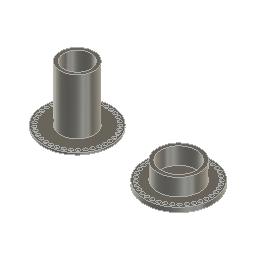
Drum (Autodesk Fusion 360 design; units mm, degrees)
part number: 2026-02-25-13-37-31-976
Autodesk Fusion 360 part; units mm, degrees
note: some values were not read from the file. Chosen so that the rebuilt part matches the saved one: which face or edge a step refers to.
sketch "Sketch1" plane through (0, 0, 0) normal (0, 0, 1) x (1, 0, 0)
  circle A0 centre (0, 0) radius 20
  circle A1 centre (-48, 22) radius 1.1
  dimension "d1" = 40
  dimension "d2" = 2.2
  constraint coincident A0.centre origin
  measures "d1" diameter of A0
  measures "d2" diameter of A1
extrude "Extrude1" add sketch "Sketch1" along normal blind 1.25 contours A0 makes body 1
sketch "Sketch2" plane through (0, 0, 1.25) normal (0, 0, 1) x (-1, 0, 0)
  circle A0 centre (0, 0) radius 20
  circle A1 centre (18, 0) radius 1.1
  circle A2 centre (17.7411, 3.042) radius 1.1
  circle A3 centre (16.9718, 5.9965) radius 1.1
  circle A4 centre (15.7143, 8.7785) radius 1.1
  circle A5 centre (14.0046, 11.308) radius 1.1
  circle A6 centre (11.8921, 13.5121) radius 1.1
  circle A7 centre (9.4375, 15.3275) radius 1.1
  circle A8 centre (6.7114, 16.702) radius 1.1
  circle A9 centre (3.7922, 17.596) radius 1.1
  circle A10 centre (0.7639, 17.9838) radius 1.1
  circle A11 centre (-2.2863, 17.8542) radius 1.1
  circle A12 centre (-5.2708, 17.211) radius 1.1
  circle A13 centre (-8.1037, 16.0727) radius 1.1
  circle A14 centre (-10.7034, 14.4719) radius 1.1
  circle A15 centre (-12.9952, 12.4549) radius 1.1
  circle A16 centre (-14.9132, 10.0795) radius 1.1
  circle A17 centre (-16.4021, 7.4142) radius 1.1
  circle A18 centre (-17.4192, 4.5356) radius 1.1
  circle A19 centre (-17.9352, 1.5265) radius 1.1
  circle A20 centre (-17.9352, -1.5265) radius 1.1
  circle A21 centre (-17.4192, -4.5356) radius 1.1
  circle A22 centre (-16.4021, -7.4142) radius 1.1
  circle A23 centre (-14.9132, -10.0795) radius 1.1
  circle A24 centre (-12.9952, -12.4549) radius 1.1
  circle A25 centre (-10.7034, -14.4719) radius 1.1
  circle A26 centre (-8.1037, -16.0727) radius 1.1
  circle A27 centre (-5.2708, -17.211) radius 1.1
  circle A28 centre (-2.2863, -17.8542) radius 1.1
  circle A29 centre (0.7639, -17.9838) radius 1.1
  circle A30 centre (3.7922, -17.596) radius 1.1
  circle A31 centre (6.7114, -16.702) radius 1.1
  circle A32 centre (9.4375, -15.3275) radius 1.1
  circle A33 centre (11.8921, -13.5121) radius 1.1
  circle A34 centre (14.0046, -11.308) radius 1.1
  circle A35 centre (15.7143, -8.7785) radius 1.1
  circle A36 centre (16.9718, -5.9965) radius 1.1
  circle A37 centre (17.7411, -3.042) radius 1.1
  dimension "d55" = 360
extrude "Extrude15" cut sketch "Sketch2" against normal blind 1.25 contours A1 | A2 | A3 | A4 | A5 | A6 | A7 | A8 | A9 | A10 | A11 | A12 | A13 | A14 | A15 | A16 | A17 | A18 | A19 | A20 | A21 | A22 | A23 | A24 | A25 | A26 | A27 | A28 | A29 | A30 | A31 | A32 | A33 | A34 | A35 | A36 | A37 bodies 1
sketch "Sketch3" plane through (0, 0, 1.25) normal (0, 0, 1) x (-1, 0, 0)
  circle A0 centre (0, 0) radius 20
  circle A1 centre (0, 0) radius 10
  circle A2 centre (18, 0) radius 1.1
  circle A3 centre (15.7143, 8.7785) radius 1.1
  circle A4 centre (6.7114, 16.702) radius 1.1
  circle A5 centre (-5.2708, 17.211) radius 1.1
  circle A6 centre (-14.9132, 10.0795) radius 1.1
  circle A7 centre (-17.9352, -1.5265) radius 1.1
  circle A8 centre (-12.9952, -12.4549) radius 1.1
  circle A9 centre (-2.2863, -17.8542) radius 1.1
  circle A10 centre (9.4375, -15.3275) radius 1.1
  circle A11 centre (16.9718, -5.9965) radius 1.1
  circle A12 centre (17.7411, -3.042) radius 1.1
  circle A13 centre (11.8921, -13.5121) radius 1.1
  circle A14 centre (0.7639, -17.9838) radius 1.1
  circle A15 centre (-10.7034, -14.4719) radius 1.1
  circle A16 centre (-17.4192, -4.5356) radius 1.1
  circle A17 centre (-16.4021, 7.4142) radius 1.1
  circle A18 centre (-8.1037, 16.0727) radius 1.1
  circle A19 centre (3.7922, 17.596) radius 1.1
  circle A20 centre (14.0046, 11.308) radius 1.1
  circle A21 centre (16.9718, 5.9965) radius 1.1
  circle A22 centre (9.4375, 15.3275) radius 1.1
  circle A23 centre (-2.2863, 17.8542) radius 1.1
  circle A24 centre (-12.9952, 12.4549) radius 1.1
  circle A25 centre (-17.9352, 1.5265) radius 1.1
  circle A26 centre (-14.9132, -10.0795) radius 1.1
  circle A27 centre (-5.2708, -17.211) radius 1.1
  circle A28 centre (6.7114, -16.702) radius 1.1
  circle A29 centre (15.7143, -8.7785) radius 1.1
  circle A30 centre (14.0046, -11.308) radius 1.1
  circle A31 centre (3.7922, -17.596) radius 1.1
  circle A32 centre (-8.1037, -16.0727) radius 1.1
  circle A33 centre (-16.4021, -7.4142) radius 1.1
  circle A34 centre (-17.4192, 4.5356) radius 1.1
  circle A35 centre (-10.7034, 14.4719) radius 1.1
  circle A36 centre (0.7639, 17.9838) radius 1.1
  circle A37 centre (11.8921, 13.5121) radius 1.1
  circle A38 centre (17.7411, 3.042) radius 1.1
  constraint coincident A0.centre A1.centre
extrude "Extrude4" add sketch "Sketch3" along normal blind 32.75 contours A1 bodies 1
sketch "Sketch4" plane through (0, 0, 34) normal (0, 0, 1) x (-1, 0, 0)
  circle A0 centre (0, 0) radius 10
  circle A1 centre (0, 0) radius 8
  constraint coincident A0.centre A1.centre
extrude "Extrude5" cut sketch "Sketch4" against normal blind 30 contours A1 bodies 1
move_body "Move1" bodies 1 to x (1, 0, 0) y (0, 1, 0) z (0, 0, 1) at (-30, 0, 0)
copy_body "CopyPasteBodies1" bodies 1 makes body 2
move_body "Move2" bodies 2 to x (1, 0, 0) y (0, 1, 0) z (0, 0, 1) at (60, 0, 0)
move_face "OffsetFaces1" offset -25 1 faces at (20.7337, 0.8943, 34) on bodies 2
delete_face "DeleteFace1" 1 faces at (20.0124, -0.4985, 3.8333) on bodies 2
sketch "Sketch5" plane through (0, 0, 1.25) normal (0, 0, 1) x (-1, 0, 0)
  circle A0 centre (-30, 0) radius 20
  circle A1 centre (-30, 0) radius 12.5
  circle A2 centre (-12, 0) radius 1.1
  circle A3 centre (-14.2857, 8.7785) radius 1.1
  circle A4 centre (-23.2886, 16.702) radius 1.1
  circle A5 centre (-35.2708, 17.211) radius 1.1
  circle A6 centre (-44.9132, 10.0795) radius 1.1
  circle A7 centre (-47.9352, -1.5265) radius 1.1
  circle A8 centre (-42.9952, -12.4549) radius 1.1
  circle A9 centre (-32.2863, -17.8542) radius 1.1
  circle A10 centre (-20.5625, -15.3275) radius 1.1
  circle A11 centre (-13.0282, -5.9965) radius 1.1
  circle A12 centre (-12.2589, -3.042) radius 1.1
  circle A13 centre (-18.1079, -13.5121) radius 1.1
  circle A14 centre (-29.2361, -17.9838) radius 1.1
  circle A15 centre (-40.7034, -14.4719) radius 1.1
  circle A16 centre (-47.4192, -4.5356) radius 1.1
  circle A17 centre (-46.4021, 7.4142) radius 1.1
  circle A18 centre (-38.1037, 16.0727) radius 1.1
  circle A19 centre (-26.2078, 17.596) radius 1.1
  circle A20 centre (-15.9954, 11.308) radius 1.1
  circle A21 centre (-13.0282, 5.9965) radius 1.1
  circle A22 centre (-20.5625, 15.3275) radius 1.1
  circle A23 centre (-32.2863, 17.8542) radius 1.1
  circle A24 centre (-42.9952, 12.4549) radius 1.1
  circle A25 centre (-47.9352, 1.5265) radius 1.1
  circle A26 centre (-44.9132, -10.0795) radius 1.1
  circle A27 centre (-35.2708, -17.211) radius 1.1
  circle A28 centre (-23.2886, -16.702) radius 1.1
  circle A29 centre (-14.2857, -8.7785) radius 1.1
  circle A30 centre (-15.9954, -11.308) radius 1.1
  circle A31 centre (-26.2078, -17.596) radius 1.1
  circle A32 centre (-38.1037, -16.0727) radius 1.1
  circle A33 centre (-46.4021, -7.4142) radius 1.1
  circle A34 centre (-47.4192, 4.5356) radius 1.1
  circle A35 centre (-40.7034, 14.4719) radius 1.1
  circle A36 centre (-29.2361, 17.9838) radius 1.1
  circle A37 centre (-18.1079, 13.5121) radius 1.1
  circle A38 centre (-12.2589, 3.042) radius 1.1
  dimension "d18" = 25
  constraint concentric A0 A1
  measures "d18" diameter of A1
extrude "Extrude6" add sketch "Sketch5" along normal blind 10 contours A1 bodies 2
sketch "Sketch6" plane through (0, 0, 11.25) normal (0, 0, 1) x (-1, 0, 0)
  circle A0 centre (-30, 0) radius 12.5
  circle A1 centre (-30, 0) radius 10.325
  dimension "d21" = 20.65
  constraint concentric A0 A1
  measures "d21" diameter of A1
sketch "Sketch8" plane through (0, 0, 11.25) normal (0, 0, 1) x (-1, 0, 0)
  circle A0 centre (-30, 0) radius 12.5
  circle A1 centre (-30, 0) radius 10.375
  dimension "d23" = 20.75
  constraint concentric A0 A1
  measures "d23" diameter of A1
extrude "Extrude7" cut sketch "Sketch8" against normal blind 10 contours A1 bodies 2
extrude "Extrude8" add 1 faces at (-31.8969, -2.8445, 4) along direction (0, 0, 1) blind 10 on bodies 1 bodies 1
sketch "Sketch9" plane through (0, 0, 0) normal (0, 0, -1) x (1, 0, 0)
  circle A0 centre (-30, 0) radius 20
  circle A1 centre (-30, 0) radius 2.75
  circle A2 centre (-48, 0) radius 1.1
  circle A3 centre (-45.7143, 8.7785) radius 1.1
  circle A4 centre (-36.7114, 16.702) radius 1.1
  circle A5 centre (-24.7292, 17.211) radius 1.1
  circle A6 centre (-15.0868, 10.0795) radius 1.1
  circle A7 centre (-12.0648, -1.5265) radius 1.1
  circle A8 centre (-17.0048, -12.4549) radius 1.1
  circle A9 centre (-27.7137, -17.8542) radius 1.1
  circle A10 centre (-39.4375, -15.3275) radius 1.1
  circle A11 centre (-46.9718, -5.9965) radius 1.1
  circle A12 centre (-47.7411, -3.042) radius 1.1
  circle A13 centre (-41.8921, -13.5121) radius 1.1
  circle A14 centre (-30.7639, -17.9838) radius 1.1
  circle A15 centre (-19.2966, -14.4719) radius 1.1
  circle A16 centre (-12.5808, -4.5356) radius 1.1
  circle A17 centre (-13.5979, 7.4142) radius 1.1
  circle A18 centre (-21.8963, 16.0727) radius 1.1
  circle A19 centre (-33.7922, 17.596) radius 1.1
  circle A20 centre (-44.0046, 11.308) radius 1.1
  circle A21 centre (-46.9718, 5.9965) radius 1.1
  circle A22 centre (-39.4375, 15.3275) radius 1.1
  circle A23 centre (-27.7137, 17.8542) radius 1.1
  circle A24 centre (-17.0048, 12.4549) radius 1.1
  circle A25 centre (-12.0648, 1.5265) radius 1.1
  circle A26 centre (-15.0868, -10.0795) radius 1.1
  circle A27 centre (-24.7292, -17.211) radius 1.1
  circle A28 centre (-36.7114, -16.702) radius 1.1
  circle A29 centre (-45.7143, -8.7785) radius 1.1
  circle A30 centre (-44.0046, -11.308) radius 1.1
  circle A31 centre (-33.7922, -17.596) radius 1.1
  circle A32 centre (-21.8963, -16.0727) radius 1.1
  circle A33 centre (-13.5979, -7.4142) radius 1.1
  circle A34 centre (-12.5808, 4.5356) radius 1.1
  circle A35 centre (-19.2966, 14.4719) radius 1.1
  circle A36 centre (-30.7639, 17.9838) radius 1.1
  circle A37 centre (-41.8921, 13.5121) radius 1.1
  circle A38 centre (-47.7411, 3.042) radius 1.1
  dimension "d28" = 5.5
  constraint concentric A0 A1
  measures "d28" diameter of A1
extrude "Extrude9" cut sketch "Sketch9" against normal blind 1.5 contours A1 bodies 1
sketch "Sketch10" plane through (0, 0, 1.5) normal (0, 0, -1) x (1, 0, 0)
  circle A0 centre (-30, 0) radius 2.75
  line L0 (-32.9795, 1.75) -> (-26.5, 1.75)
  line L1 (-26.5, 1.75) -> (-26.5, -1.75)
  line L2 (-26.5, -1.75) -> (-32.9795, -1.75)
  line L3 (-32.9795, -1.75) -> (-32.9795, 1.75)
  dimension "d31" = 3.5
  dimension "d32" = 1.75
  constraint horizontal L0
  constraint vertical L1
  constraint horizontal L2
  constraint vertical L3
  measures "d31" distance of L0.start L2.end
  measures "d32" distance of A0.centre L0
extrude "Extrude10" cut sketch "Sketch10" against normal blind 7 contours A0 L0 L2 bodies 1
sketch "Sketch11" plane through (0, 0, 0) normal (0, 0, -1) x (1, 0, 0)
  circle A0 centre (30, 0) radius 20
  circle A1 centre (18, 0) radius 4
  circle A2 centre (12, 0) radius 1.1
  circle A3 centre (14.2857, 8.7785) radius 1.1
  circle A4 centre (23.2886, 16.702) radius 1.1
  circle A5 centre (35.2708, 17.211) radius 1.1
  circle A6 centre (44.9132, 10.0795) radius 1.1
  circle A7 centre (47.9352, -1.5265) radius 1.1
  circle A8 centre (42.9952, -12.4549) radius 1.1
  circle A9 centre (32.2863, -17.8542) radius 1.1
  circle A10 centre (20.5625, -15.3275) radius 1.1
  circle A11 centre (13.0282, -5.9965) radius 1.1
  circle A12 centre (12.2589, -3.042) radius 1.1
  circle A13 centre (18.1079, -13.5121) radius 1.1
  circle A14 centre (29.2361, -17.9838) radius 1.1
  circle A15 centre (40.7034, -14.4719) radius 1.1
  circle A16 centre (47.4192, -4.5356) radius 1.1
  circle A17 centre (46.4021, 7.4142) radius 1.1
  circle A18 centre (38.1037, 16.0727) radius 1.1
  circle A19 centre (26.2078, 17.596) radius 1.1
  circle A20 centre (15.9954, 11.308) radius 1.1
  circle A21 centre (13.0282, 5.9965) radius 1.1
  circle A22 centre (20.5625, 15.3275) radius 1.1
  circle A23 centre (32.2863, 17.8542) radius 1.1
  circle A24 centre (42.9952, 12.4549) radius 1.1
  circle A25 centre (47.9352, 1.5265) radius 1.1
  circle A26 centre (44.9132, -10.0795) radius 1.1
  circle A27 centre (35.2708, -17.211) radius 1.1
  circle A28 centre (23.2886, -16.702) radius 1.1
  circle A29 centre (14.2857, -8.7785) radius 1.1
  circle A30 centre (15.9954, -11.308) radius 1.1
  circle A31 centre (26.2078, -17.596) radius 1.1
  circle A32 centre (38.1037, -16.0727) radius 1.1
  circle A33 centre (46.4021, -7.4142) radius 1.1
  circle A34 centre (47.4192, 4.5356) radius 1.1
  circle A35 centre (40.7034, 14.4719) radius 1.1
  circle A36 centre (29.2361, 17.9838) radius 1.1
  circle A37 centre (18.1079, 13.5121) radius 1.1
  circle A38 centre (12.2589, 3.042) radius 1.1
  dimension "d36" = 8
  measures "d36" diameter of A1
extrude "Extrude11" add 1 faces at (25.7728, 14.8426, 1.25) along direction (0, 0, 1) blind 1.5 on bodies 2 bodies 2
extrude "Extrude12" add 1 faces at (18.2549, 0.621, 11.25) along direction (0, 0, 1) blind 1.5 on bodies 2 bodies 2
extrude "Extrude13" add 1 faces at (26.4369, -2.4293, 1.25) along direction (0, 0, 1) blind 1.5 on bodies 2 bodies 2
extrude "Extrude14" cut sketch "Sketch11" against normal blind 2.2 contours A1 bodies 2
sketch "Sketch12" plane through (0, 0, 0) normal (0, 0, -1) x (1, 0, 0)
  circle A0 centre (18, 0) radius 4
  circle A1 centre (12, 0) radius 1.1
  circle A2 centre (30, 0) radius 20
  circle A3 centre (30, 0) radius 1.5
  circle A4 centre (14.2857, 8.7785) radius 1.1
  circle A5 centre (23.2886, 16.702) radius 1.1
  circle A6 centre (35.2708, 17.211) radius 1.1
  circle A7 centre (44.9132, 10.0795) radius 1.1
  circle A8 centre (47.9352, -1.5265) radius 1.1
  circle A9 centre (42.9952, -12.4549) radius 1.1
  circle A10 centre (32.2863, -17.8542) radius 1.1
  circle A11 centre (20.5625, -15.3275) radius 1.1
  circle A12 centre (13.0282, -5.9965) radius 1.1
  circle A13 centre (12.2589, -3.042) radius 1.1
  circle A14 centre (18.1079, -13.5121) radius 1.1
  circle A15 centre (29.2361, -17.9838) radius 1.1
  circle A16 centre (40.7034, -14.4719) radius 1.1
  circle A17 centre (47.4192, -4.5356) radius 1.1
  circle A18 centre (46.4021, 7.4142) radius 1.1
  circle A19 centre (38.1037, 16.0727) radius 1.1
  circle A20 centre (26.2078, 17.596) radius 1.1
  circle A21 centre (15.9954, 11.308) radius 1.1
  circle A22 centre (13.0282, 5.9965) radius 1.1
  circle A23 centre (20.5625, 15.3275) radius 1.1
  circle A24 centre (32.2863, 17.8542) radius 1.1
  circle A25 centre (42.9952, 12.4549) radius 1.1
  circle A26 centre (47.9352, 1.5265) radius 1.1
  circle A27 centre (44.9132, -10.0795) radius 1.1
  circle A28 centre (35.2708, -17.211) radius 1.1
  circle A29 centre (23.2886, -16.702) radius 1.1
  circle A30 centre (14.2857, -8.7785) radius 1.1
  circle A31 centre (15.9954, -11.308) radius 1.1
  circle A32 centre (26.2078, -17.596) radius 1.1
  circle A33 centre (38.1037, -16.0727) radius 1.1
  circle A34 centre (46.4021, -7.4142) radius 1.1
  circle A35 centre (47.4192, 4.5356) radius 1.1
  circle A36 centre (40.7034, 14.4719) radius 1.1
  circle A37 centre (29.2361, 17.9838) radius 1.1
  circle A38 centre (18.1079, 13.5121) radius 1.1
  circle A39 centre (12.2589, 3.042) radius 1.1
  dimension "d49" = 3
  constraint concentric A2 A3
  measures "d49" diameter of A3
extrude "Extrude16" add sketch "Sketch12" along normal blind 5 contours A3 bodies 2
fillet "Fillet1" radius 1 1 edges at (28.6015, 0.5424, -5) on bodies 2
move_body "Move3" bodies 2 to x (-1, 0, 0) y (0, 1, 0) z (0, 0, -1) at (60, 0, 13)
move_body "Move4" bodies 2 to x (1, 0, 0) y (0, 1, 0) z (0, 0, 1) at (-60, 0, 24)
sketch "Sketch7" plane through (0, 0, 11.25) normal (0, 0, 1) x (-1, 0, 0)
  circle A0 centre (-30, 0) radius 12
  circle A1 centre (-30, 0) radius 10.375
  dimension "d22" = 20.75
  constraint concentric A0 A1
  measures "d22" diameter of A1
move_body "Move5" bodies 2 to x (-1, 0, 0) y (0, 1, 0) z (0, 0, -1) at (0, 0, 37.5)
equation "d32 = ( 3.5 / 2 ) * 1 mm"
